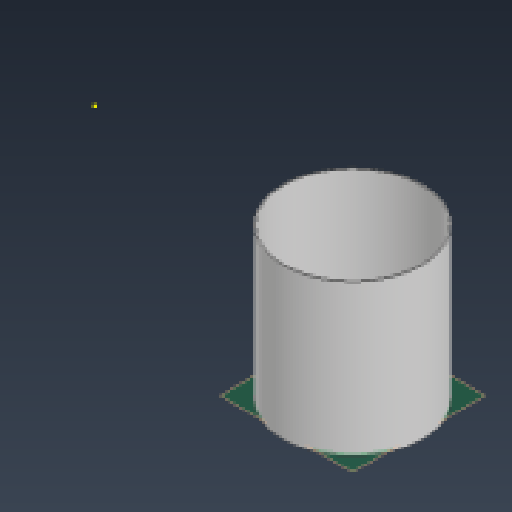
# Autodesk Inventor part: doWylewanka
Saved by Autodesk Inventor 2023 (Build 270158000, 158)
## iProperties
Created: 2025-03-26
Part Number: doWylewanka
Material: Generic
Document SubType Name: Modeling
Designer: szymo
Density: 1 g/cm^3
Appearance: Default
Author: szymo
Autodesk Inventor part; units mm, degrees
ref_plane "YZ Plane" through (0, 0, 0) normal (1, 0, 0) x (0, 1, 0)
ref_plane "XZ Plane" through (0, 0, 0) normal (0, 1, 0) x (-1, 0, 0)
ref_plane "XY Plane" through (0, 0, 0) normal (0, 0, 1) x (1, 0, 0)
sketch "Sketch1" plane through (0, 0, 0) normal (0, 1, 0) x (-1, 0, 0)
  point P0 (0, 0)
ref_plane "Work Plane1" through (96.0134, -42.5085, 2.0528) normal (0, -1, 0) x (1, 0, 0)
sketch "Sketch2" plane through (96.0134, -42.5085, 2.0528) normal (0, -1, 0) x (1, 0, 0)
  arc A0 (-14.4004, -10.7994) -> (-7.7362, -10.3996) centre (-11.2003, -8.3996) ccw projected
  arc A1 (-16.5528, -7.0714) -> (-14.4004, -10.7994) centre (0, 0) ccw projected
  arc A2 (-12.8744, -1.5) -> (-16.5528, -7.0714) centre (-12.8744, -5.5) ccw projected
  line L0 (-8.6603, -1.5) -> (-12.8744, -1.5) projected
  arc A3 (-5.6292, -6.75) -> (-8.6603, -1.5) centre (-8.6603, -5) ccw projected
  line L1 (-7.7362, -10.3996) -> (-5.6292, -6.75) projected
  circle A4 centre (0, 0) radius 22 projected
  arc A5 (-8.6603, 1.5) -> (-5.6292, 6.75) centre (-8.6603, 5) ccw projected
  line L2 (-12.8744, 1.5) -> (-8.6603, 1.5) projected
  arc A6 (-16.5528, 7.0714) -> (-12.8744, 1.5) centre (-12.8744, 5.5) ccw projected
  arc A7 (-14.4004, 10.7994) -> (-16.5528, 7.0714) centre (0, 0) ccw projected
  arc A8 (-7.7362, 10.3996) -> (-14.4004, 10.7994) centre (-11.2003, 8.3996) ccw projected
  line L3 (-5.6292, 6.75) -> (-7.7362, 10.3996) projected
  arc A9 (-3.0311, 8.25) -> (3.0311, 8.25) centre (0, 10) ccw projected
  line L4 (-5.1382, 11.8996) -> (-3.0311, 8.25) projected
  arc A10 (-2.1524, 17.8709) -> (-5.1382, 11.8996) centre (-1.6741, 13.8996) ccw projected
  arc A11 (2.1524, 17.8709) -> (-2.1524, 17.8709) centre (0, 0) ccw projected
  arc A12 (5.1382, 11.8996) -> (2.1524, 17.8709) centre (1.6741, 13.8996) ccw projected
  line L5 (3.0311, 8.25) -> (5.1382, 11.8996) projected
  arc A13 (14.4004, 10.7994) -> (7.7362, 10.3996) centre (11.2003, 8.3996) ccw projected
  arc A14 (16.5528, 7.0714) -> (14.4004, 10.7994) centre (0, 0) ccw projected
  arc A15 (12.8744, 1.5) -> (16.5528, 7.0714) centre (12.8744, 5.5) ccw projected
  line L6 (8.6603, 1.5) -> (12.8744, 1.5) projected
  arc A16 (5.6292, 6.75) -> (8.6603, 1.5) centre (8.6603, 5) ccw projected
  line L7 (7.7362, 10.3996) -> (5.6292, 6.75) projected
  arc A17 (8.6603, -1.5) -> (5.6292, -6.75) centre (8.6603, -5) ccw projected
  line L8 (12.8744, -1.5) -> (8.6603, -1.5) projected
  arc A18 (16.5528, -7.0714) -> (12.8744, -1.5) centre (12.8744, -5.5) ccw projected
  arc A19 (14.4004, -10.7994) -> (16.5528, -7.0714) centre (0, 0) ccw projected
  arc A20 (7.7362, -10.3996) -> (14.4004, -10.7994) centre (11.2003, -8.3996) ccw projected
  line L9 (5.6292, -6.75) -> (7.7362, -10.3996) projected
  arc A21 (-5.1382, -11.8996) -> (-2.1524, -17.8709) centre (-1.6741, -13.8996) ccw projected
  line L10 (-3.0311, -8.25) -> (-5.1382, -11.8996) projected
  arc A22 (3.0311, -8.25) -> (-3.0311, -8.25) centre (0, -10) ccw projected
  line L11 (5.1382, -11.8996) -> (3.0311, -8.25) projected
  arc A23 (2.1524, -17.8709) -> (5.1382, -11.8996) centre (1.6741, -13.8996) ccw projected
  arc A24 (-2.1524, -17.8709) -> (2.1524, -17.8709) centre (0, 0) ccw projected
  arc A25 (-2.2605, 3.3) -> (-2.2605, -3.3) centre (0, 0) ccw projected
  line L12 (2.2605, 3.3) -> (-2.2605, 3.3) projected
  arc A26 (2.2605, -3.3) -> (2.2605, 3.3) centre (0, 0) ccw projected
  line L13 (-2.2605, -3.3) -> (2.2605, -3.3) projected
  circle A27 centre (0, 0) radius 25.5
  point P0 (-96.0134, -2.0528)
  dimension "d0" = 51
  constraints: 1 centre point, 1 coincident
  measures "d0" diameter of A27
extrude "Extrusion1" add sketch "Sketch2" along normal blind 1 contours A1 A2 L0 A3 L1 A0 | A4 | L2 A6 A7 A8 L3 A5 | L4 A10 A11 A12 L5 A9 | A14 A15 L6 A16 L7 A13 | L8 A18 A19 A20 L9 A17 | L10 A22 L11 A23 A24 A21 | L12 A26 L13 A25 | A27
sketch "Sketch3" plane through (96.0134, -42.5085, 2.0528) normal (0, 1, 0) x (1, 0, 0)
  circle A0 centre (0, 0) radius 25.5 projected
  circle A1 centre (0, 0) radius 25
  point P0 (-96.0134, 2.0528)
  dimension "d3" = 50
  constraints: 1 centre point, 1 coincident
  measures "d3" diameter of A1
extrude "Extrusion2" add sketch "Sketch3" along normal blind 54
body "Solid1"
